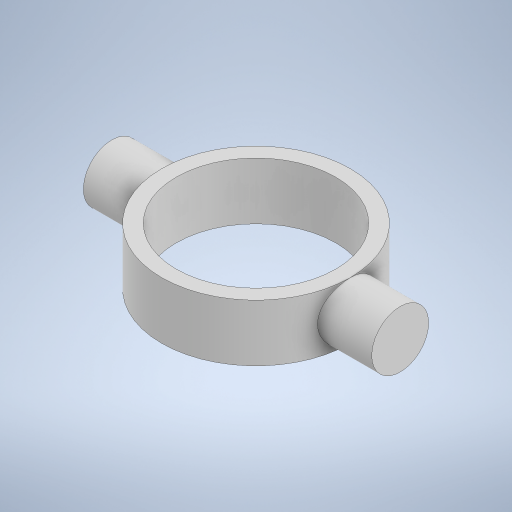
# Autodesk Inventor part: anillo central
Saved by Autodesk Inventor 2024 (Build 280153000, 153)
## iProperties
Created: 2024-04-03
Part Number: anillo central
Material: Generic
Document SubType Name: Modeling
Designer: compu
Density: 1 g/cm^3
Appearance: Default
Author: compu
Autodesk Inventor part; units mm, degrees
ref_plane "YZ Plane" through (0, 0, 0) normal (1, 0, 0) x (0, 1, 0)
ref_plane "XZ Plane" through (0, 0, 0) normal (0, 1, 0) x (-1, 0, 0)
sketch "Sketch6" plane through (0, 0, 0) normal (0, 1, 0) x (-1, 0, 0)
  circle A0 centre (0, 0) radius 4
  circle A1 centre (0, 0) radius 11.2
  circle A2 centre (0, 0) radius 14
  circle A3 centre (0, 0) radius 13.25
  line L0 (4, 13.4164) -> (-4, 13.4164)
  line L1 (19.6, 0) -> (-19.6, 0) projected
  point P0 (13.25, 0)
  point P1 (-13.25, 0)
  point P2 (-14, 0)
  point P3 (14, 0)
  dimension "d13" = 8
  dimension "d14" = 22.4
  dimension "d15" = 28
  dimension "d16" = 26.5
  dimension "d17" = 8
  constraints: 4 centre point, 4 coincident, 2 end point, 2 point on circle, 1 horizontal, 1 parallel
  measures "d13" diameter of A0
  measures "d14" diameter of A1
  measures "d15" diameter of A2
  measures "d16" diameter of A3
  measures "d17" distance of L0.start L0.end
extrude "Extrusion7" add sketch "Sketch6" along normal blind 8 contours L1 A3 A1 | A1 L1 A3
sketch "Sketch9" plane through (0, 8, 0) normal (0, 1, 0) x (1, 0, 0)
  circle A0 centre (0, 0) radius 13.25 projected
  line L0 (-18.55, 0) -> (18.55, 0) projected
  point P0 (13.25, 0)
  constraints: 1 horizontal alignment, 1 point on line, 1 other
ref_plane "Work Plane3" through (13.25, 8, 0) normal (1, 0, 0) x (0, 1, 0)
sketch "Sketch10" plane through (13.25, 8, 0) normal (1, 0, 0) x (0, 1, 0)
  line L0 (-9.6, 0) -> (1.6, 0) projected
  line L1 (-9.6, 0) -> (1.6, 0) projected
  line L2 (-8, 13.25) -> (0, 13.25) projected
  line L3 (-8, -13.25) -> (0, -13.25) projected
  line L4 (0, -13.25) -> (0, 13.25) projected
  line L5 (-8, -13.25) -> (-8, 13.25) projected
  line L6 (0, -13.25) -> (-8, 13.25)
  circle A0 centre (-4, 0) radius 4
  point P0 (-8, 0)
  dimension "d30" = 8
  constraints: 2 end point, 1 centre point, 1 midpoint
  measures "d30" diameter of A0
extrude "Extrusion8" add sketch "Sketch10" against normal up to surface contours A0 L6 L0 | L0 L6 A0 | L6 A0 L0 | L0 A0 L6
extrude "Extrusion9" add sketch "Sketch10" along normal blind 7 contours A0 L6 L0 | L0 L6 A0 | L6 A0 L0 | L0 A0 L6
pattern_circular "Circular Pattern3" count 2 over 360 about axis through (0, 0, 0) along (0, 1, 0) of "Extrusion8", "Extrusion9"
body "Solid3"
